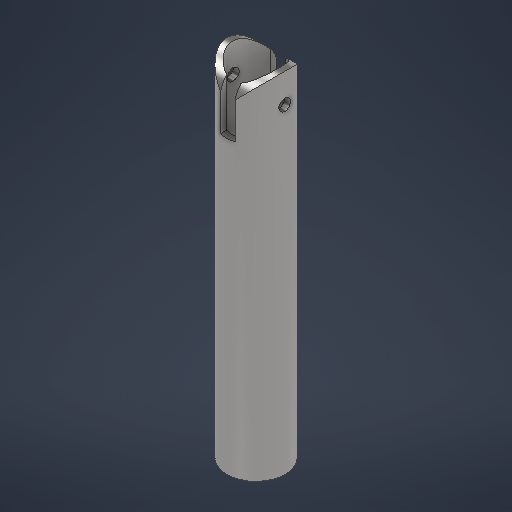
# Autodesk Inventor part: Shaft
Saved by Autodesk Inventor 2026.2 (Build 302298010, 298A)
## iProperties
Created: 2026-04-02
Part Number: Shaft
Material: Stainless Steel
Document SubType Name: Modeling
Designer: piete
Density: 8 g/cm^3
Appearance: Semi-Polished
Author: piete
Autodesk Inventor part; units mm, degrees
ref_plane "YZ Plane" through (0, 0, 0) normal (1, 0, 0) x (0, 1, 0)
ref_plane "XZ Plane" through (0, 0, 0) normal (0, 1, 0) x (-1, 0, 0)
ref_plane "XY Plane" through (0, 0, 0) normal (0, 0, 1) x (1, 0, 0)
sketch "Sketch1" plane through (0, 0, 0) normal (0, 1, 0) x (-1, 0, 0)
  circle A0 centre (0, 0) radius 5
  circle A1 centre (0, 0) radius 4
  dimension "d0" = 10
  dimension "d1" = 8
  constraints: 2 centre point, 2 coincident
  measures "d0" diameter of A0
  measures "d1" diameter of A1
extrude "Extrusion1" add sketch "Sketch1" along normal blind 60
sketch "Sketch2" plane through (0, 0, 0) normal (1, 0, 0) x (0, 1, 0)
  circle A0 centre (55, 0) radius 5
  line L0 (60, 4) -> (60, -4) projected
  circle A1 centre (55, 0) radius 1
  line L1 (55, -5) -> (60, -5)
  line L2 (0, -5) -> (60, -5) projected
  line L3 (60, -5) -> (60, 5) projected
  line L4 (55, 5) -> (60, 5)
  line L5 (60, 5) -> (60, -5)
  point P0 (0, 0)
  point P1 (60, 0)
  point P2 (60, 0)
  dimension "d4" = 10
  dimension "d5" = 5
  dimension "d6" = 0
  dimension "d7" = 2
  constraints: 6 end point, 2 centre point, 2 point on circle, 2 tangent, 1 coincident, 1 collinear, 1 midpoint, 1 point on line
  measures "d4" diameter of A0
  measures "d5" distance from line of L0 A0.centre
  measures "d6" vertical distance of point (60, 0) A0.centre
  measures "d7" diameter of A1
extrude "Extrusion2" cut sketch "Sketch2" along normal through all both and the other way through all contours L0 L3 L1 A0 | A0 L4 L3 L0 | A1
sketch "Sketch3" plane through (0, 0, 0) normal (0, 0, 1) x (1, 0, 0)
  line L0 (-1.25, 60) -> (1.25, 60)
  line L1 (1.25, 60) -> (1.25, 50)
  line L2 (1.25, 50) -> (-1.25, 50)
  line L3 (-1.25, 50) -> (-1.25, 60)
  line L4 (-5, 0) -> (-5, 60) projected
  line L5 (5, 60) -> (-5, 60) projected
  point P0 (0, 0)
  point P1 (0, 50)
  dimension "d10" = 2.5
  dimension "d11" = 10
  dimension "d12" = 0
  dimension "d13" = 5
  constraints: 8 end point, 2 parallel, 1 horizontal, 1 midpoint, 1 perpendicular
  measures "d10" distance of L1.end L2.end
  measures "d11" distance of L0.end L1.end
  measures "d12" distance between parallel lines of L5 L0
  measures "d13" distance from line of L4 point (0, 50)
extrude "Extrusion3" cut sketch "Sketch3" along normal through all both and the other way through all
body "Solid1"
